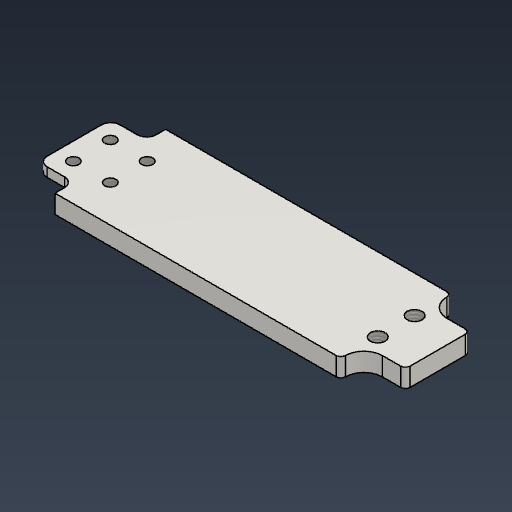
# Autodesk Inventor part: Kicker Eisen
Saved by Autodesk Inventor 2023.1 (Build 271208000, 208)
## iProperties
Part Number: Kicker Eisen
Material: Stahl, unlegiert
Document SubType Name: Modeling
Designer: rYan
Mass: 51.6105 g
Surface Area: 42.6729 cm^2
Volume: 6.57458 cm^3
Density: 7.85 g/cm^3
Appearance: Stahl
Author: rYan
Autodesk Inventor part; units mm, degrees
ref_plane "YZ Plane" through (0, 0, 0) normal (1, 0, 0) x (0, 1, 0)
ref_plane "XZ Plane" through (0, 0, 0) normal (0, 1, 0) x (-1, 0, 0)
ref_plane "XY Plane" through (0, 0, 0) normal (0, 0, 1) x (1, 0, 0)
sketch "Skizze1" plane through (0, 0, 0) normal (0, 0, 1) x (1, 0, 0)
  line L0 (0, 12) -> (62, 12)
  line L1 (62, -12) -> (0, -12)
  line L2 (0, -12) -> (0, 12)
  line L3 (-14.2, 0) -> (85.2, 0) projected
  line L4 (62, -7) -> (71, -7)
  line L5 (71, -7) -> (71, 7)
  line L6 (71, 7) -> (62, 7)
  line L7 (62, 12) -> (62, 7)
  line L8 (62, -7) -> (62, -12)
  point P0 (0, 0)
  dimension "d0" = 24
  dimension "d1" = 62
  dimension "d29" = 14
  dimension "d30" = 9
  constraints: 16 end point, 4 parallel, 3 perpendicular, 2 horizontal, 1 collinear, 1 midpoint, 2 other
  measures "d0" distance of L1.end L0.start
  measures "d1" distance of L0.start L0.end
  measures "d29" distance of L4.end L5.end
  measures "d30" distance of L5.end L6.end
extrude "Extrusion1" add sketch "Skizze1" along normal blind 4
sketch "Skizze5" plane through (0, 0, 0) normal (0, 0, -1) x (-1, 0, 0)
  line L0 (0, -12) -> (0, 12) construction
  line L1 (-85.2, 0) -> (14.2, 0) construction
  line L2 (0, 12) -> (0, -12) projected
  line L3 (0, -8) -> (-6, -8)
  line L4 (-8, -6) -> (-8, 6)
  line L5 (-6, 8) -> (0, 8)
  line L6 (0, 8) -> (0, -8)
  arc A0 (-8, -6) -> (-6, -8) centre (-6, -6) ccw
  arc A1 (-6, 8) -> (-8, 6) centre (-6, 6) ccw
  point P0 (0, 0)
  dimension "d37" = 2
  dimension "d38" = 4
  dimension "d39" = 8
  constraints: 8 end point, 4 point on circle, 4 tangent, 2 centre point, 2 parallel, 1 equal radius, 1 horizontal, 1 perpendicular, 1 point on line, 2 other
  measures "d37" radius of A0
  measures "d38" distance from line of L0.start L3
  measures "d39" distance between parallel lines of L0 L4
extrude "Extrusion3" cut sketch "Skizze5" against normal blind 2
sketch "Skizze6" plane through (0, 0, 4) normal (0, 0, 1) x (1, 0, 0)
  line L0 (0, 12) -> (0, -12) construction
  line L1 (-24.0571, 0) -> (86.8428, 0) construction
  line L2 (0, 7.9) -> (-5.8, 7.9)
  line L3 (-7.8, 5.9) -> (-7.8, -5.9)
  line L4 (-5.8, -7.9) -> (0, -7.9)
  line L5 (0, -7.9) -> (0, 7.9)
  arc A0 (-5.8, 7.9) -> (-7.8, 5.9) centre (-5.8, 5.9) ccw
  arc A1 (-7.8, -5.9) -> (-5.8, -7.9) centre (-5.8, -5.9) ccw
  point P0 (0, 0)
  dimension "d42" = 2
  dimension "d43" = 4.1
  dimension "d44" = 7.8
  constraints: 8 end point, 4 point on circle, 4 tangent, 2 centre point, 2 parallel, 1 equal radius, 1 horizontal, 1 perpendicular, 1 point on line, 2 other
  measures "d42" radius of A0
  measures "d43" distance from line of L0.start L2
  measures "d44" distance between parallel lines of L0 L3
extrude "Extrusion4" add sketch "Skizze6" against normal blind 2
sketch "Skizze2" plane through (0, 0, 4) normal (0, 0, 1) x (1, 0, 0)
  line L0 (62, 12) -> (0, 12) projected
  line L1 (0, 12) -> (0, -12) projected
  line L2 (0, 12) -> (4, 12)
  line L3 (4, 12) -> (4, -12)
  line L4 (4, -12) -> (0, -12)
  line L5 (0, -12) -> (0, 12)
  point P0 (0, 0)
  dimension "d4" = 4
  constraints: 8 end point, 2 parallel, 1 horizontal, 1 perpendicular, 1 point on line
  measures "d4" distance between parallel lines of L1 L3
extrude "Extrusion2" [suppressed]
sketch "Skizze3" plane through (0, 0, 2) normal (0, 0, 1) x (1, 0, 0)
  line L0 (0, 16.8) -> (0, -16.8) projected
  line L1 (-15, 0) -> (90, 0) projected
  point P0 (0, 0)
  point P1 (2, 0)
  dimension "d7" = 2
  constraints: 1 point on line
  measures "d7" distance from line of L0 point (2, 0)
hole "Bohrung1" [suppressed]
pattern_linear "Rechteckige Anordnung1" [suppressed]
sketch "Skizze4" plane through (0, 0, 4) normal (0, 0, 1) x (1, 0, 0)
  line L0 (-14.2, 0) -> (85.2, 0) projected
  line L1 (62, -12) -> (62, 12) projected
  line L2 (71, -7) -> (71, 7) construction
  point P0 (0, 0)
  point P1 (62, 4)
  point P2 (62, -4)
  dimension "d31" = 8
  dimension "d36" = 0
  constraints: 1 symmetric about line
  measures "d31" distance of point (62, -4) point (62, 4)
  measures "d36" distance from line of point (62, -4) L1
hole "Bohrung2" at (62, -4, 4) at (62, 4, 4) direction (0, 0, -1) diameter 3.242 end through all thread size "M4x0.7" class "6H" standard "ISO Metric profile"
fillet "Rundung1" radius 4 2 edges at (62, -7, 2) (62, 7, 2)
fillet "Rundung2" radius 1 4 edges at (62, -12, 2) (62, 12, 2) (71, -7, 2) (71, 7, 2)
sketch "Skizze7" plane through (0, 0, 0) normal (0, 0, 1) x (1, 0, 0)
  line L0 (-4, -4) -> (4, -4) construction
  line L1 (4, -4) -> (4, 4) construction
  line L2 (4, 4) -> (-4, 4) construction
  line L3 (-4, 4) -> (-4, -4) construction
  line L4 (0, 5.6) -> (0, -5.6) construction
  line L5 (-5.6, 0) -> (5.6, 0) construction
  point P0 (0, 0)
  dimension "d48" = 8
  dimension "d49" = 8
  constraints: 8 end point, 4 coincident, 2 parallel, 1 horizontal, 1 perpendicular, 2 other
  measures "d48" distance of L0.start L0.end
  measures "d49" distance of L2.end L0.start
hole "Bohrung3" at (4, -4, 0) at (4, 4, 0) at (-4, 4, 0) at (-4, -4, 0) direction (0, 0, 1) diameter 2.459 end through all thread size "M3x0.5" class "6H" standard "ISO Metric profile"
fillet "Rundung3" radius 2 4 edges at (0, -8, 1) (0, 8, 1) (0, 7.9, 3) (0, -7.9, 3)
